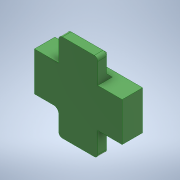
# Autodesk Inventor part: 071_0100_Base
Saved by Autodesk Inventor 2020 (Build 240168000, 168)
## iProperties
Created: 2018-07-06
Part Number: 071_0100_Base
Material: Generic
Document SubType Name: Modeling
Designer: deniz
Density: 1 g/cm^3
Appearance: Default
Author: deniz
Autodesk Inventor part; units mm, degrees
ref_plane "YZ Plane" through (0, 0, 0) normal (1, 0, 0) x (0, 1, 0)
ref_plane "XZ Plane" through (0, 0, 0) normal (0, 1, 0) x (-1, 0, 0)
sketch "Sketch1" plane through (0, 0, 0) normal (0, 1, 0) x (-1, 0, 0)
  line L0 (0, 0) -> (45, 0)
  line L1 (45, 0) -> (45, -45)
  line L2 (45, -45) -> (0, -45)
  line L3 (0, -45) -> (0, 0)
  line L4 (32.5, 0) -> (32.5, -12.5)
  line L5 (32.5, -12.5) -> (45, -12.5)
  line L6 (32.5, -32.5) -> (32.5, -45)
  line L7 (32.5, -32.5) -> (45, -32.5)
  line L8 (12.5, -32.5) -> (0, -32.5)
  line L9 (12.5, -32.5) -> (12.5, -45)
  line L10 (12.5, -12.5) -> (12.5, 0)
  line L11 (12.5, -12.5) -> (0, -12.5)
  line L12 (32.5, -3) -> (12.5, -3)
  line L13 (12.5, -12.5) -> (32.5, -12.5)
  line L14 (32.5, -12.5) -> (32.5, -32.5) construction
  line L15 (32.5, -32.5) -> (12.5, -32.5)
  line L16 (12.5, -32.5) -> (12.5, -12.5) construction
  line L17 (12.5, -12.5) -> (32.5, -32.5) construction
  line L18 (32.5, -12.5) -> (12.5, -32.5) construction
  circle A0 centre (22.5, -22.5) radius 13
  line L19 (32.5, -42) -> (12.5, -42)
  line L20 (42, -32.5) -> (42, -12.5)
  line L21 (3, -32.5) -> (3, -12.5)
  dimension "d2" = 20
  dimension "d8" = 20
  dimension "d9" = 45
  dimension "d10" = 12.5
  dimension "d11" = 45
  dimension "d12" = 12.5
  dimension "d13" = 3
  dimension "d16" = 26
  dimension "d24" = 3
  dimension "d25" = 3
  dimension "d26" = 3
  dimension "d30" = 12.5
  constraints: 44 end point, 23 point on line, 8 perpendicular, 5 parallel, 2 horizontal, 1 centre point, 1 collinear, 1 midpoint, 1 vertical
  measures "d2" distance between parallel lines of L7 L5
  measures "d8" distance between parallel lines of L9 L6
  measures "d9" distance of L1.end L2.end
  measures "d10" distance of L10.start L11.end
  measures "d11" distance between parallel lines of L0 L2
  measures "d12" distance between parallel lines of L0 L11
  measures "d13" distance between parallel lines of L0 L12
  measures "d16" diameter of A0
  measures "d24" distance between parallel lines of L2 L19
  measures "d25" distance between parallel lines of L21 L3
  measures "d26" distance between parallel lines of L1 L20
  measures "d30" distance of L4.end L5.end
extrude "Extrusion1Base" add sketch "Sketch1" along normal blind 6 contours L0 L4 L12 L10 | L11 L21 L8 L3 | L12 L4 L13 A0 L10 | L11 L13 A0 L15 L8 L21 | L1 L7 L20 L5 | L5 L20 L7 L15 A0 L13 | A0 L13 | L13 A0 L15 | L9 L19 L6 L2 | L15 A0 L6 L19 L9 | L15 A0
fillet "OrientationFillet1" radius 2.7 1 edges at (-32.5, 3, -32.5)
extrude "Grips" add sketch "Sketch1" along normal blind 12 contours L11 L21 L8 L3 | L11 L13 A0 L15 L8 L21 | L1 L7 L20 L5 | L5 L20 L7 L15 A0 L13 | L13 A0 L15
fillet "Fillet2" radius 1.8 4 edges at (-32.5, 3, 0) (-12.5, 3, 0) (-32.5, 3, -45) (-12.5, 3, -45)
sketch "Sketch3" plane through (-22.5, 12, -22.5) normal (0, 1, 0) x (1, 0, 0)
  circle A0 centre (0, 0) radius 3.5
  point P0 (22.5, -22.5)
  dimension "d20" = 7
  constraints: 1 centre point, 1 coincident
  measures "d20" diameter of A0
extrude "Extrusion5" cut sketch "Sketch3" against normal blind 6
ref_plane "Work Plane1" through (-12.5, 0, -12.5) normal (-0.7071068, 0, 0.7071068) x (0, 1, 0)
sketch "Sketch5" plane through (0, 12, 0) normal (0, 1, 0) x (1, 0, 0)
  circle A0 centre (-22.5, 22.5) radius 3.5 projected
  line L0 (-45, 12.5) -> (0, 12.5) projected
  line L1 (0, 12.5) -> (0, 32.5) projected
  line L2 (0, 32.5) -> (-45, 32.5) projected
  line L3 (-45, 32.5) -> (-45, 12.5) projected
  arc A1 (-14.3, 0) -> (-12.5, 1.8) centre (-14.3, 1.8) ccw projected
  line L4 (-12.5, 1.8) -> (-12.5, 12.5) projected
  line L5 (-12.5, 12.5) -> (-32.5, 12.5) projected
  line L6 (-32.5, 12.5) -> (-32.5, 1.8) projected
  arc A2 (-32.5, 1.8) -> (-30.7, 0) centre (-30.7, 1.8) ccw projected
  line L7 (-30.7, 0) -> (-14.3, 0) projected
  line L8 (-25.5788, 24.1646) -> (-33.9142, 32.5)
  line L9 (-22.5, 22.5) -> (-32.5, 32.5)
  point P0 (0, 0)
  point P1 (-24.9749, 24.9749)
  dimension "d37" = 45
  dimension "d40" = 1
  constraints: 4 end point, 2 point on line, 2 other
  measures "d37" angle of L2 L9
  measures "d40" distance between parallel lines of L9 L8
revolve "Revolution2" cut sketch "Sketch5" angle 360 about axis through (-22.5, 12, -22.5) along (-0.7071068, 0, -0.7071068) contours L8 L2 L9 A0
chamfer "Chamfer2" distance 1.5 angle 45 2 edges at (-23.3585, 12, -19.1069) (-20.7078, 12, -25.5063)
chamfer "Chamfer3" distance 1.5 angle 45 17 edges at (-22.5, 12, -12.5) (-45, 12, -22.5) (-39.4571, 12, -32.5) (0, 12, -22.5) (-22.5, 6, -12.5) (-23.85, 6, -32.5) (-31.9728, 6, -0.5272) (-32.5, 6, -7.15) (-22.5, 6, 0) (-13.0272, 6, -0.5272) (-12.5, 6, -7.15) (-22.5, 6, -45) (-31.9728, 6, -44.4728) (-32.5, 6, -39.2) (-33.2908, 6, -33.2908) (-13.0272, 6, -44.4728) (-12.5, 6, -37.85)
equation "\"d8\" = d2"
equation "\"d24\" = d13"
equation "\"d25\" = d13"
equation "\"d26\" = d13"
body "Solid1"
